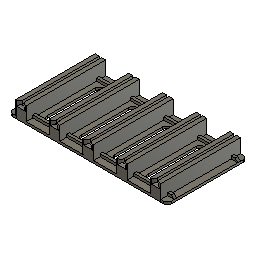
card_guide (Autodesk Fusion 360 design; units mm, degrees)
Autodesk Fusion 360 part; units mm, degrees
sketch "Sketch1" plane through (0, 0, 0) normal (0, 1, 0) x (1, 0, 0)
  line L0 (0, 0) -> (8, 0)
  line L1 (8, 0) -> (8, -60)
  line L2 (0.6, -60) -> (0, -60)
  line L3 (0, -60) -> (0, 0)
  line L4 (3.1, -57.5) -> (3.1, 0)
  line L5 (4.9, 0) -> (4.9, -57.5)
  arc A0 (0.6, -60) -> (3.1, -57.5) centre (0.6, -57.5) ccw
  line L6 (8, -60) -> (7.4, -60)
  arc A1 (4.9, -57.5) -> (7.4, -60) centre (7.4, -57.5) ccw
  line L7 (7.4, -60) -> (0, -60)
  line L8 (30.3, 0) -> (30.3, -57.5)
  line L9 (33.4, -60) -> (32.8, -60)
  line L10 (26, -60) -> (25.4, -60)
  arc A2 (26, -60) -> (28.5, -57.5) centre (26, -57.5) ccw
  line L11 (25.4, -60) -> (25.4, 0)
  line L12 (25.4, 0) -> (33.4, 0)
  line L13 (33.4, 0) -> (33.4, -60)
  arc A3 (30.3, -57.5) -> (32.8, -60) centre (32.8, -57.5) ccw
  line L14 (32.8, -60) -> (25.4, -60)
  line L15 (28.5, -57.5) -> (28.5, 0)
  line L16 (55.7, 0) -> (55.7, -57.5)
  line L17 (58.8, -60) -> (58.2, -60)
  line L18 (51.4, -60) -> (50.8, -60)
  arc A4 (51.4, -60) -> (53.9, -57.5) centre (51.4, -57.5) ccw
  line L19 (50.8, -60) -> (50.8, 0)
  line L20 (50.8, 0) -> (58.8, 0)
  line L21 (58.8, 0) -> (58.8, -60)
  arc A5 (55.7, -57.5) -> (58.2, -60) centre (58.2, -57.5) ccw
  line L22 (58.2, -60) -> (50.8, -60)
  line L23 (53.9, -57.5) -> (53.9, 0)
  line L24 (81.1, 0) -> (81.1, -57.5)
  line L25 (84.2, -60) -> (83.6, -60)
  line L26 (76.8, -60) -> (76.2, -60)
  arc A6 (76.8, -60) -> (79.3, -57.5) centre (76.8, -57.5) ccw
  line L27 (76.2, -60) -> (76.2, 0)
  line L28 (76.2, 0) -> (84.2, 0)
  line L29 (84.2, 0) -> (84.2, -60)
  arc A7 (81.1, -57.5) -> (83.6, -60) centre (83.6, -57.5) ccw
  line L30 (83.6, -60) -> (76.2, -60)
  line L31 (79.3, -57.5) -> (79.3, 0)
  line L32 (106.5, 0) -> (106.5, -57.5)
  line L33 (109.6, -60) -> (109, -60)
  line L34 (102.2, -60) -> (101.6, -60)
  arc A8 (102.2, -60) -> (104.7, -57.5) centre (102.2, -57.5) ccw
  line L35 (101.6, -60) -> (101.6, 0)
  line L36 (101.6, 0) -> (109.6, 0)
  line L37 (109.6, 0) -> (109.6, -60)
  arc A9 (106.5, -57.5) -> (109, -60) centre (109, -57.5) ccw
  line L38 (109, -60) -> (101.6, -60)
  line L39 (104.7, -57.5) -> (104.7, 0)
  line L40 (8, 0) -> (25.4, 0)
  line L41 (33.4, 0) -> (50.8, 0)
  line L42 (58.8, 0) -> (76.2, 0)
  line L43 (84.2, 0) -> (101.6, 0)
  line L44 (8, -60) -> (25.4, -60)
  line L45 (33.4, -60) -> (50.8, -60)
  line L46 (58.8, -60) -> (76.2, -60)
  line L47 (84.2, -60) -> (101.6, -60)
  line L48 (15, -9) -> (18.4, -9)
  line L49 (21.4, -12) -> (21.4, -48)
  line L50 (18.4, -51) -> (15, -51)
  line L51 (12, -48) -> (12, -12)
  arc A10 (15, -9) -> (12, -12) centre (15, -12) ccw
  arc A11 (21.4, -12) -> (18.4, -9) centre (18.4, -12) ccw
  arc A12 (12, -48) -> (15, -51) centre (15, -48) ccw
  arc A13 (18.4, -51) -> (21.4, -48) centre (18.4, -48) ccw
  line L52 (0, 0) -> (-2, 0)
  line L53 (-5, -3) -> (-5, -57)
  line L54 (-2, -60) -> (0.6, -60)
  arc A14 (-2, 0) -> (-5, -3) centre (-2, -3) ccw
  arc A15 (-2, 0) -> (-5, -3) centre (-2, -3) ccw
  arc A16 (-5, -57) -> (-2, -60) centre (-2, -57) ccw
  line L55 (46.8, -12) -> (46.8, -48)
  line L56 (37.4, -48) -> (37.4, -12)
  line L57 (43.8, -51) -> (40.4, -51)
  arc A17 (43.8, -51) -> (46.8, -48) centre (43.8, -48) ccw
  arc A18 (46.8, -12) -> (43.8, -9) centre (43.8, -12) ccw
  arc A19 (40.4, -9) -> (37.4, -12) centre (40.4, -12) ccw
  line L58 (40.4, -9) -> (43.8, -9)
  arc A20 (37.4, -48) -> (40.4, -51) centre (40.4, -48) ccw
  line L59 (72.2, -12) -> (72.2, -48)
  line L60 (62.8, -48) -> (62.8, -12)
  line L61 (69.2, -51) -> (65.8, -51)
  arc A21 (69.2, -51) -> (72.2, -48) centre (69.2, -48) ccw
  arc A22 (72.2, -12) -> (69.2, -9) centre (69.2, -12) ccw
  arc A23 (65.8, -9) -> (62.8, -12) centre (65.8, -12) ccw
  line L62 (65.8, -9) -> (69.2, -9)
  arc A24 (62.8, -48) -> (65.8, -51) centre (65.8, -48) ccw
  line L63 (97.6, -12) -> (97.6, -48)
  line L64 (88.2, -48) -> (88.2, -12)
  line L65 (94.6, -51) -> (91.2, -51)
  arc A25 (94.6, -51) -> (97.6, -48) centre (94.6, -48) ccw
  arc A26 (97.6, -12) -> (94.6, -9) centre (94.6, -12) ccw
  arc A27 (91.2, -9) -> (88.2, -12) centre (91.2, -12) ccw
  line L66 (91.2, -9) -> (94.6, -9)
  arc A28 (88.2, -48) -> (91.2, -51) centre (91.2, -48) ccw
  line L67 (109.6, 0) -> (111.6, 0)
  line L68 (114.6, -3) -> (114.6, -57)
  line L69 (111.6, -60) -> (109.6, -60)
  arc A29 (114.6, -3) -> (111.6, 0) centre (111.6, -3) ccw
  arc A30 (111.6, -60) -> (114.6, -57) centre (111.6, -57) ccw
  point P0 (25.4, 0)
  point P1 (50.8, 0)
  point P2 (76.2, 0)
  point P3 (101.6, 0)
  point P4 (114.6, 0)
  point P5 (4, -9)
  point P6 (4, -51)
  point P7 (18, -56)
  point P8 (105.6, -9)
  point P9 (105.6, -51)
  dimension "d1" = 8
  dimension "d2" = 60
  dimension "d7" = 3.1
  dimension "d8" = 3.1
  dimension "d9" = 2.5
  dimension "d10" = 2.5
  dimension "d13" = 25.4
  dimension "d14" = 0
  dimension "d15" = 9
  dimension "d16" = 9
  dimension "d17" = 4
  dimension "d18" = 4
  dimension "d19" = 3
  dimension "d20" = 3
  dimension "d21" = 3
  dimension "d22" = 3
  dimension "d23" = 3
  dimension "d24" = 3
  dimension "d27" = 25.4
  dimension "d28" = 0
  dimension "d29" = 5
  dimension "d30" = 3
  dimension "d31" = 3
  dimension "d43" = 4
  dimension "d44" = 4
  constraint horizontal L0
  constraint vertical L1
  constraint horizontal L2
  constraint vertical L3
  constraint coincident L0.start L3.end
  constraint perpendicular L2 L4
  constraint coincident L0 L5.start
  constraint perpendicular L2 L5
  constraint coincident L1.end L2
  constraint tangent L2 A0
  constraint tangent L4 A0
  constraint tangent L5 A1
  constraint tangent L6 A1
  constraint tangent A1 L7
  constraint coincident P0 L11.end
  constraint coincident P1 L19.end
  constraint coincident P2 L27.end
  constraint coincident P3 L35.end
  constraint horizontal L48
  constraint vertical L49
  constraint horizontal L50
  constraint vertical L51
  constraint tangent L48 A10
  constraint tangent L51 A10
  constraint tangent L48 A11
  constraint tangent L49 A11
  constraint tangent L51 A12
  constraint tangent L50 A12
  constraint tangent L49 A13
  constraint tangent L50 A13
  constraint perpendicular L3 L52
  constraint perpendicular L0 L53
  constraint tangent A0 L54
  constraint tangent L52 A14
  constraint tangent L53 A14
  constraint coincident L52 A14.start
  constraint coincident L53 A14.end
  constraint tangent L52 A15
  constraint tangent L53 A15
  constraint equal A14 A15
  constraint tangent L54 A16
  constraint tangent L53 A16
  constraint perpendicular L37 L67
  constraint perpendicular L67 L68
  constraint coincident P4 L67
  constraint coincident P4 L68
  constraint tangent L67 A29
  constraint tangent L68 A29
  constraint tangent L69 A30
  constraint tangent L68 A30
  measures "d1" distance of L0.start L0.end
  measures "d2" distance of L0.start L2.end
  measures "d7" distance of L3 L4
  measures "d8" distance of L1 L5
  measures "d9" radius of A0
  measures "d10" radius of A1
  measures "d15" distance of L40 L48
  measures "d16" distance of L44 L50
  measures "d17" distance of L1 L51
  measures "d18" distance of L11 L49
  measures "d19" radius of A10
  measures "d20" radius of A11
  measures "d21" radius of A12
  measures "d22" radius of A13
  measures "d23" radius of A14
  measures "d24" radius of A16
  measures "d29" distance of L36.end P4
  measures "d30" radius of A29
  measures "d31" radius of A30
  measures "d43" distance of L35 P8
  measures "d44" distance of L35 P9
extrude "Extrude1" add sketch "Sketch1" against normal blind 1.8
extrude "Extrude2" add sketch "Sketch1" along normal blind 8 contours L0 L4 L5 A0 A1 L7 | L8 A2 L12 A3 L14 L15 | L16 A4 L20 A5 L22 L23 | L24 A6 L28 A7 L30 L31 | L32 A8 L36 A9 L38 L39
extrude "Extrude3" add sketch "Sketch1" along normal blind 10.4 contours L0 L2 L3 L4 A0 L7 L54 | L0 L1 L5 L6 A1 | L10 A2 L11 L12 L14 L15 | L8 L9 L12 L13 A3 | L18 A4 L19 L20 L22 L23 | L16 L17 L20 L21 A5 | L26 A6 L27 L28 L30 L31 | L24 L25 L28 L29 A7 | L34 A8 L35 L36 L38 L39 | L32 L33 L36 L37 A9
fillet "Fillet1" radius 1.5 1 edges at (4, 8, 60)
fillet "Fillet1" radius 1.5 1 edges at (29.4, 8, 60)
fillet "Fillet1" radius 1.5 1 edges at (54.8, 8, 60)
fillet "Fillet1" radius 1.5 1 edges at (80.2, 8, 60)
fillet "Fillet1" radius 1.5 1 edges at (105.6, 8, 60)
sketch "Sketch2" plane through (0, 0, 0) normal (0, 1, 0) x (1, 0, 0)
box "BoxPrimitive1" add length 2 width 119.6 height 2 placed x (0, 0, -1) y (-1, 0, 0) z (0, 1, 0) at (114.6, 0, 55)
box "BoxPrimitive2" add length 2 width 119.6 height 2 placed x (0, 0, 1) y (1, 0, 0) z (0, 1, 0) at (-5, 0, 5)
hole "Hole1" at (4, 0, 51) at (4, 0, 9) at (105.6, 0, 51) at (105.6, 0, 9) direction (0, 1, 0) diameter 5 depth 5 tip angle 118
hole "Hole2" at (4, 0, 51) at (4, 0, 9) at (105.6, 0, 9) at (105.6, 0, 51) direction (0, -1, 0) diameter 5 depth 5 tip angle 118
chamfer "Chamfer1" distance 2 angle 45 1 edges at (-5, 2, 54)
chamfer "Chamfer2" distance 2 angle 45 3 edges at (-5, 2, 6) (114.6, 2, 54) (114.6, 2, 6)
